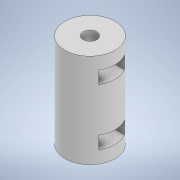
# Autodesk Inventor part: axe_millieu
Saved by Autodesk Inventor 2020 (Build 240168000, 168)
## iProperties
Created: 2020-06-16
Part Number: axe_millieu
Material: Generic
Document SubType Name: Modeling
Designer: Admin
Density: 1 g/cm^3
Appearance: Default
Author: Admin
Autodesk Inventor part; units mm, degrees
ref_plane "YZ Plane" through (0, 0, 0) normal (1, 0, 0) x (0, 1, 0)
ref_plane "XZ Plane" through (0, 0, 0) normal (0, 1, 0) x (-1, 0, 0)
ref_plane "XY Plane" through (0, 0, 0) normal (0, 0, 1) x (1, 0, 0)
sketch "Sketch6" plane through (0, 0, 0) normal (0, 1, 0) x (-1, 0, 0)
  line L0 (4, 4) -> (-4, 4)
  line L1 (-4, 4) -> (-4, -4)
  line L2 (-4, -4) -> (4, -4)
  line L3 (4, -4) -> (4, 4)
  point P0 (0, 0)
  dimension "d24" = 8
  dimension "d25" = 8
  dimension "d26" = 4
  dimension "d27" = 4
  constraints: 8 end point, 2 parallel, 1 horizontal, 1 perpendicular
  measures "d24" distance of L2.end L0.start
  measures "d25" distance of L1.end L2.end
  measures "d26" distance from line of L3 point (0, 0)
  measures "d27" distance from line of point (0, 0) L2
extrude "Extrusion6" add sketch "Sketch6" along normal blind 15
sketch "Sketch7" plane through (4, 0, 4) normal (1, 0, 0) x (0, 0, -1)
  line L0 (1.95, 4) -> (6.05, 4)
  line L1 (6.05, 4) -> (6.05, 2)
  line L2 (6.05, 2) -> (1.95, 2)
  line L3 (1.95, 2) -> (1.95, 4)
  line L4 (0, 0) -> (0, 15) projected
  line L5 (0, 0) -> (8, 0) projected
  line L6 (1.95, 13) -> (6.05, 13)
  line L7 (6.05, 13) -> (6.05, 11)
  line L8 (6.05, 11) -> (1.95, 11)
  line L9 (1.95, 11) -> (1.95, 13)
  line L10 (0, 15) -> (8, 15) projected
  point P0 (4, 0)
  dimension "d30" = 4.1
  dimension "d31" = 2
  dimension "d32" = 1.95
  dimension "d33" = 2
  dimension "d37" = 4.1
  dimension "d38" = 2
  dimension "d39" = 1.95
  dimension "d40" = 2
  constraints: 16 end point, 4 parallel, 2 horizontal, 2 perpendicular
  measures "d30" distance of L0.start L0.end
  measures "d31" distance of L0.end L1.end
  measures "d32" distance between parallel lines of L4 L3
  measures "d33" distance between parallel lines of L5 L2
  measures "d37" distance of L6.start L6.end
  measures "d38" distance of L6.end L7.end
  measures "d39" distance between parallel lines of L4 L9
  measures "d40" distance between parallel lines of L10 L6
extrude "Extrusion7" cut sketch "Sketch7" against normal through all
fillet "Fillet1" radius 4 4 edges at (4, 7.5, 4) (-4, 7.5, 4) (4, 7.5, -4) (-4, 7.5, -4)
sketch "Sketch8" plane through (0, 15, 0) normal (0, 1, 0) x (1, 0, 0)
  circle A0 centre (0, 0) radius 1.1
  dimension "d41" = 2.2
  constraints: 1 centre point, 1 coincident
  measures "d41" diameter of A0
extrude "Extrusion8" cut sketch "Sketch8" against normal through all
body "Solid2"
